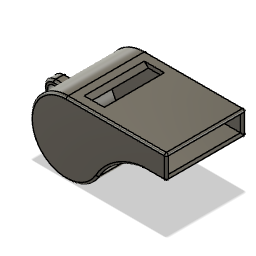
baba bday gift pt1 v1 (Autodesk Fusion 360 design; units mm, degrees)
Autodesk Fusion 360 part; units mm, degrees
sketch "Sketch1" plane through (0, 0, 0) normal (0, 0, 1) x (1, 0, 0)
  circle A0 centre (0, 0) radius 9
  line L0 (0, 9) -> (25, 9)
  line L1 (25, 9) -> (25, 3)
  line L2 (25, 3) -> (19, 3)
  arc A1 (19, 3) -> (7.8189, -4.457) centre (20.8503, -11.8854) ccw
  dimension "d1" = 18
  dimension "d2" = 25
  dimension "d3" = 6
  dimension "d4" = 6
  dimension "d5" = 15
  constraint coincident A0.centre origin
  constraint horizontal L0
  constraint coincident A0 L0.start
  constraint tangent A0 L0
  constraint perpendicular L0 L1
  constraint perpendicular L1 L2
  constraint coincident A0 A1.end
  constraint tangent A0 A1
  measures "d1" diameter of A0
  measures "d2" distance of L0.start L0.end
  measures "d3" distance of L0.end L1.end
  measures "d4" distance of L1.end L2.end
  measures "d5" radius of A1
extrude "Extrude1" add sketch "Sketch1" along normal mid plane 20
shell "Shell1" thickness 1 removed faces 1 at (25, 7, 3.3333)
sketch "Sketch2" plane through (0, 0, 0) normal (0, 0, 1) x (1, 0, 0)
  line L0 (0, 9) -> (25, 9)
  line L1 (0, 8) -> (25, 8)
  line L2 (2, 9) -> (3, 8)
  line L3 (2, 9) -> (1.4972, 9) construction
  line L4 (7, 9) -> (6, 8)
  line L5 (7, 9) -> (6.4972, 9) construction
  dimension "d9" = 45
  dimension "d10" = 135
  dimension "d11" = 3
  dimension "d12" = 2
  constraint horizontal L3
  constraint coincident L0 L2.start
  constraint coincident L1 L2.end
  constraint horizontal L5
  constraint coincident L0 L4.start
  constraint coincident L1 L4.end
  measures "d9" angle of L2 L3
  measures "d10" angle of L4 L5
  measures "d11" distance of L2.end L4.end
  measures "d12" distance of L0.start L2.start
extrude "Extrude2" cut sketch "Sketch2" along normal mid plane 15
sketch "Sketch3" plane through (0, 0, 0) normal (0, 0, 1) x (1, 0, 0)
  line L0 (-11.6458, 2.5) -> (-8.6458, 2.5)
  line L1 (-8.6458, 2.5) -> (-8.6458, -2.5)
  line L2 (-8.6458, -2.5) -> (-11.6458, -2.5)
  line L3 (-11.6458, -2.5) -> (-11.6458, 2.5)
  arc A0 (0, 9) -> (7.8189, -4.457) centre (0, 0) ccw
  arc A1 (-11.6458, 2.5) -> (-11.6458, -2.5) centre (-11.6458, 0) ccw
  circle A2 centre (-11.6458, 0) radius 1.5
  dimension "d15" = 3
  dimension "d16" = 5
  dimension "d17" = 3
  constraint horizontal L0
  constraint vertical L1
  constraint horizontal L2
  constraint vertical L3
  constraint coincident L0.end A0
  constraint coincident L1.end A0
  constraint tangent L0 A1
  constraint concentric A1 A2
  measures "d15" distance of L0.start L0.end
  measures "d16" distance of L0.start L2.end
  measures "d17" diameter of A2
extrude "Extrude3" add sketch "Sketch3" along normal mid plane 3 contours L0 L2 L3 A0 A2 | L3 A1 A2
fillet "Fillet1" radius 0.5 18 edges at (12.5, 9, 10) (-7.7818, -4.5214, 10) (12.5275, 0.5938, 10) (25, 9, 0) (25, 6, 10) (22, 3, 10) (25, 3, 0) (25, 6, -10) (12.5275, 0.5938, -10) (-7.7818, -4.5214, -10) (12.5, 9, -10) (22, 3, -10) (-10.1458, 2.5, 1.5) (-14.1458, 0, 1.5) (-10.1458, -2.5, 1.5) (-10.1458, -2.5, -1.5) (-14.1458, 0, -1.5) (-10.1458, 2.5, -1.5)
chamfer "Chamfer1" distance 0.5 angle 45 4 edges at (25, 4, 0) (25, 6, -9) (25, 8, 0) (25, 6, 9)
